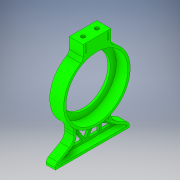
# Autodesk Inventor part: Inductor Legs
Saved by Autodesk Inventor 2018 (Build 220112000, 112)
## iProperties
Created: 2017-12-03
Part Number: Inductor Legs
Material: Generic
Document SubType Name: Modeling
Designer: xdlea
Density: 1 g/cm^3
Appearance: Default(2)
legHeight: 2.694 in
Author: xdlea
Autodesk Inventor part; units mm, degrees
ref_plane "YZ Plane" through (0, 0, 0) normal (1, 0, 0) x (0, 1, 0)
ref_plane "XZ Plane" through (0, 0, 0) normal (0, 1, 0) x (-1, 0, 0)
ref_plane "XY Plane" through (0, 0, 0) normal (0, 0, 1) x (1, 0, 0)
sketch "Sketch - PVC Pipe" plane through (0, 0, 0) normal (1, 0, 0) x (0, 1, 0)
  circle A0 centre (0, 0) radius 21.0693
  circle A1 centre (0, 0) radius 17.0656
sketch "Leg Sketch" plane through (0, 0, 0) normal (1, 0, 0) x (0, 1, 0)
  arc A0 (-22.8699, 0) -> (-20.0097, -11.0744) centre (0, 0) ccw
  circle A1 centre (0, 0) radius 17.0656 projected
  circle A2 centre (0, 0) radius 21.0693 construction
  line L0 (-19.0195, 12.7) -> (-27.5927, 12.7)
  line L1 (-27.5927, 12.7) -> (-34.925, 25.4)
  line L2 (-34.925, 25.4) -> (-38.1, 25.4)
  line L3 (-38.1, 25.4) -> (-38.1, -25.4)
  line L4 (-38.1, -25.4) -> (-34.925, -25.4)
  line L5 (-34.925, -25.4) -> (-27.5927, -12.7)
  line L6 (-27.5927, -12.7) -> (-19.0195, -12.7)
  circle A3 centre (0, 0) radius 21.2443
  line L7 (-22.5998, 9.4488) -> (-34.8488, 1.9089)
  line L8 (-34.8488, 1.9089) -> (-34.8488, 9.4488)
  line L9 (-34.8488, 9.4488) -> (-22.5998, 9.4488)
  line L10 (-30.4083, 11.0744) -> (-34.8488, 18.7656)
  line L11 (-34.8488, 18.7656) -> (-34.8488, 11.0744)
  line L12 (-34.8488, 11.0744) -> (-30.4083, 11.0744)
  line L13 (-23.4734, 7.0022) -> (-34.8488, 0)
  line L14 (-34.8488, 0) -> (-24.4955, 0)
  arc A4 (-23.4734, 7.0022) -> (-24.4955, 0) centre (0, 0) ccw
  arc A5 (-19.0195, 12.7) -> (-20.0097, 11.0744) centre (0, 0) ccw
  arc A6 (-19.0195, -12.7) -> (-19.0195, 12.7) centre (0, 0) ccw
  line L15 (-28.5312, 11.0744) -> (-35.8635, 23.7744)
  line L16 (-35.8635, 23.7744) -> (-36.4744, 23.7744)
  line L17 (-36.4744, 23.7744) -> (-36.4744, -23.7744)
  line L18 (-36.4744, -23.7744) -> (-35.8635, -23.7744)
  line L19 (-35.8635, -23.7744) -> (-28.5312, -11.0744)
  line L20 (-20.0097, 11.0744) -> (-28.5312, 11.0744)
  line L21 (-20.0097, -11.0744) -> (-28.5312, -11.0744)
  arc A7 (-20.0097, 11.0744) -> (-22.8699, 0) centre (0, 0) ccw
  arc A8 (-20.0097, -11.0744) -> (-19.0195, -12.7) centre (0, 0) ccw
  line L22 (20.792, 9.525) -> (30.317, 9.525)
  line L23 (30.317, 9.525) -> (30.317, -9.525)
  line L24 (30.317, -9.525) -> (20.792, -9.525)
  line L25 (20.792, -9.525) -> (20.792, 9.525) construction
  line L26 (21.0693, 0) -> (21.0693, -14.5729) construction
  line L27 (29.5042, 7.8994) -> (24.4242, 7.8994)
  line L28 (24.4242, 7.8994) -> (24.4242, 7.2446)
  line L29 (24.4242, 7.2446) -> (29.5042, 7.2446)
  line L30 (29.5042, 7.2446) -> (29.5042, 7.8994)
  line L31 (29.5042, -7.2446) -> (24.4242, -7.2446)
  line L32 (24.4242, -7.2446) -> (24.4242, -7.8994)
  line L33 (24.4242, -7.8994) -> (29.5042, -7.8994)
  line L34 (29.5042, -7.8994) -> (29.5042, -7.2446)
  line L35 (-51.7834, 0) -> (44.0004, 0) projected
  point P0 (25.5545, 9.525)
  dimension "d2" = 25.4
  dimension "d3" = 3.175
  dimension "d4" = 30
  dimension "d5" = 0.175
  dimension "d6" = 1.6256
  dimension "d7" = 50.8
  dimension "d13" = 38.1
  dimension "d21" = 1.6256
  dimension "d23" = 1.6256
  dimension "d25" = 1.6256
  dimension "d26" = 1.6256
  dimension "d27" = 1.6256
  dimension "d28" = 1.6256
  dimension "d29" = 1.6256
  dimension "d50" = 19.05
  dimension "d51" = 9.525
  dimension "d61" = 5.08
  dimension "d62" = 0.6548
  dimension "d63" = 1.6256
  dimension "d64" = 1.6256
  dimension "d65" = 0.8128
  dimension "d66" = 68.417
  constraints: 71 end point, 15 point on circle, 10 parallel, 9 perpendicular, 7 centre point, 5 horizontal, 4 collinear, 4 vertical, 3 point on line, 2 coincident, 1 concentric, 1 horizontal alignment, 1 midpoint, 9 other
  measures "d2" distance between parallel lines of L6 L0
  measures "d3" distance of L1.end L2.end
  measures "d4" angle of L3 L1
  measures "d6" radial gap between concentric circles of A0 A3
  measures "d7" distance of L2.end L3.end
  measures "d13" distance from line of A4.centre L3
  measures "d21" distance between parallel lines of L3 L17
  measures "d23" distance between parallel lines of L0 L20
  measures "d25" distance between parallel lines of L20 L9
  measures "d26" distance between parallel lines of L15 L10
  measures "d27" distance between parallel lines of L17 L11
  measures "d28" distance between parallel lines of L13 L7
  measures "d29" radial gap between concentric circles of A4 A5
  measures "d50" distance of L22.end L23.end
  measures "d51" distance of L23.end L24.end
  measures "d61" distance of L27.start L27.end
  measures "d62" distance of L29.end L27.start
  measures "d63" distance between parallel lines of L22 L27
  measures "d64" distance between parallel lines of L24 L33
  measures "d65" distance between parallel lines of L30 L23
  measures "d66" distance between parallel lines of L3 L23
extrude "Sheath" add sketch "Leg Sketch" along normal blind 9.525 contours L35 A3 A6 A8 A0 | A7 A5 A6 L35 A3
extrude "Leg" add sketch "Leg Sketch" along normal blind 6.35 contours L35 A4 L13 L17 L16 L15 L20 A7 | A0 L21 L19 L18 L17 L35 L14 | A8 L6 L5 L4 L3 L35 L17 L18 L19 L21 | L20 L15 L16 L17 L35 L3 L2 L1 L0 A5 | L14 L13 A4 | L7 L8 L9 | L12 L11 L10
extrude "Tube Stop" add sketch "Leg Sketch" along normal blind 1.6256 contours L35 A1 A3 | A3 L35 A1
extrude "Inner Carve" cut sketch "Leg Sketch" against normal blind 4.7244 from surface at 6.35 contours L35 A4 L13 L17 L16 L15 L20 A7 | A0 L21 L19 L18 L17 L35 L14 | L14 L13 A4 | L7 L8 L9 | L12 L11 L10
extrude "Truss" cut sketch "Leg Sketch" along normal up to next contours L14 L13 A4 | L7 L8 L9 | L12 L11 L10
mirror "Mirror1" about plane through (0, 0, 0) normal (0, 0, 1) of "Truss"
fillet "Fillet1" radius 6.35 6 edges at (3.175, -19.0195, 12.7) (3.175, -27.5927, 12.7) (3.175, -19.0195, -12.7) (3.175, -27.5927, -12.7) (3.9878, -28.5312, 11.0744) (3.9878, -28.5312, -11.0744)
fillet "Fillet2" radius 3.175 2 edges at (3.175, -34.925, 25.4) (3.175, -34.925, -25.4)
fillet "Fillet3" radius 0.4064 15 edges at (0.8128, -34.8488, -18.7656) (0.8128, -34.8488, -11.0744) (0.8128, -30.4083, -11.0744) (0.8128, -34.8488, -9.4488) (0.8128, -34.8488, -1.9089) (0.8128, -22.5998, -9.4488) (0.8128, -23.4734, -7.0022) (0.8128, -23.4734, 7.0022) (0.8128, -34.8488, 0) (0.8128, -34.8488, 1.9089) (0.8128, -34.8488, 9.4488) (0.8128, -22.5998, 9.4488) (0.8128, -30.4083, 11.0744) (0.8128, -34.8488, 11.0744) (0.8128, -34.8488, 18.7656)
extrude "Extrusion9" add sketch "Leg Sketch" along normal up to surface (9.525 mm away) contours A6 L35 L23 L24 | L22 L23 L35 A6
fillet "Fillet5" radius 3.175 2 edges at (4.7625, 20.792, 9.525) (4.7625, 20.792, -9.525)
sketch "Sketch3" plane through (0, 30.317, 9.525) normal (0, 1, 0) x (1, 0, 0)
  circle A0 centre (4.7625, 14.2875) radius 1.397
  circle A1 centre (4.7625, 4.7625) radius 1.397
  line L0 (11.43, 9.525) -> (-1.905, 9.525) projected
  point P0 (0, 9.525)
  dimension "d55" = 2.794
  dimension "d56" = 4.7625
  dimension "d57" = 4.7625
  constraints: 2 centre point, 1 other
  measures "d55" diameter of A0
  measures "d56" distance from line of L0 A0.centre
  measures "d57" horizontal distance of A0.centre point (0, 9.525)
extrude "Extrusion10" cut sketch "Sketch3" against normal up to next
derived "Conductive Rail.ipt"
equation "\"d61\" = springSteelWidth"
equation "\"d62\" = springSteelThickness"
equation "\"d64\" = d63"
equation "\"clothesHangerDia\" = 0.8128"
equation "\"railWidth\" = 13.05"
equation "\"railHeight\" = 11.25295"
equation "\"legHeight\" = 68.41699"
equation "\"springSteelWidth\" = 5.08"
equation "\"springSteelThickness\" = 0.6548"
body "Solid1"
